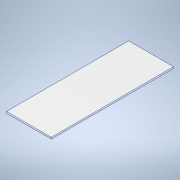
# Autodesk Inventor part: AxisY
Saved by Autodesk Inventor 2022 (Build 260153000, 153)
## iProperties
Created: 2023-08-15
Part Number: AxisY
Material: Aluminum 6061
Document SubType Name: Modeling
Designer: Kippi
Mass: 2808 g
Surface Area: 2736 cm^2
Volume: 1040 cm^3
Density: 2.7 g/cm^3
Appearance: Aluminum - Flat
Author: Kippi
Autodesk Inventor part; units mm, degrees
ref_plane "YZ Plane" through (0, 0, 0) normal (1, 0, 0) x (0, 1, 0)
ref_plane "XZ Plane" through (0, 0, 0) normal (0, 1, 0) x (-1, 0, 0)
ref_plane "XY Plane" through (0, 0, 0) normal (0, 0, 1) x (1, 0, 0)
sketch "Sketch1" plane through (0, 0, 0) normal (0, 1, 0) x (-1, 0, 0)
  line L0 (115.3846, 192.3077) -> (-104.6154, 192.3077)
  line L1 (-104.6154, 192.3077) -> (-104.6154, -407.6923)
  line L2 (-104.6154, -407.6923) -> (115.3846, -407.6923)
  line L3 (115.3846, -407.6923) -> (115.3846, 192.3077)
  point P0 (0, 0)
  dimension "d0" = 220
  dimension "d1" = 600
  constraints: 8 end point, 2 parallel, 1 horizontal, 1 perpendicular
  measures "d0" distance of L0.start L0.end
  measures "d1" distance of L2.end L0.start
extrude "Extrusion1" add sketch "Sketch1" along normal blind 8
body "Solid1"
